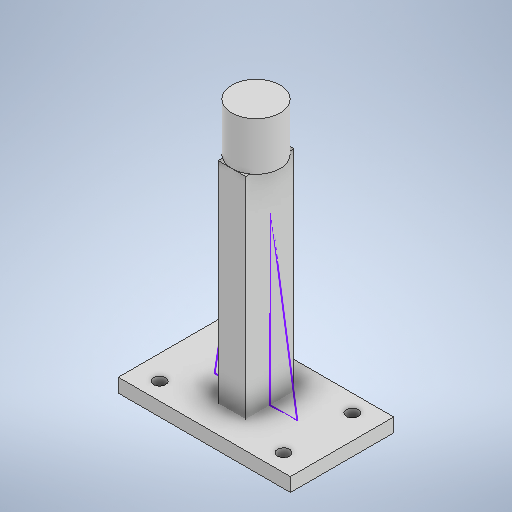
# Autodesk Inventor part: Stuetze_v2
Saved by Autodesk Inventor 2025 (Build 290162000, 162)
## iProperties
Created: 2026-06-23
Part Number: Stuetze_v2
Material: Generisch
Document SubType Name: Modeling
Designer: GemmiDad-GBSE
Density: 1 g/cm^3
Appearance: Vorgabe
Author: GemmiDad-GBSE
Autodesk Inventor part; units mm, degrees
ref_plane "YZ Plane" through (0, 0, 0) normal (1, 0, 0) x (0, 1, 0)
ref_plane "XZ Plane" through (0, 0, 0) normal (0, 1, 0) x (-1, 0, 0)
sketch "Skizze1" plane through (0, 0, 0) normal (0, 0, 1) x (1, 0, 0)
  line L0 (-25, -15) -> (25, -15)
  line L1 (25, -15) -> (25, 15)
  line L2 (25, 15) -> (-25, 15)
  line L3 (-25, 15) -> (-25, -15)
  constraints: 8 end point, 2 parallel, 1 horizontal, 1 perpendicular
extrude "Extrusion1" add sketch "Skizze1" along normal blind 4
sketch "Skizze2" plane through (0, 0, 0) normal (0, 0, 1) x (1, 0, 0)
  line L0 (-4, -7) -> (4, -7)
  line L1 (4, -7) -> (4, 7)
  line L2 (4, 7) -> (-4, 7)
  line L3 (-4, 7) -> (-4, -7)
  constraints: 8 end point, 2 parallel, 1 horizontal, 1 perpendicular
extrude "Extrusion2" add sketch "Skizze2" along normal blind 65 separate body
ref_plane "Arbeitsebene1" through (0, 0, 65) normal (0, 0, 1) x (1, 0, 0)
sketch "Skizze3" plane through (0, 0, 65) normal (0, 0, 1) x (1, 0, 0)
  circle A0 centre (0, 0) radius 7
  constraints: 1 centre point
extrude "Extrusion3" add sketch "Skizze3" along normal blind 14 separate body
sketch "Skizze4" plane through (0, 0, 0) normal (0, 1, 0) x (-1, 0, 0)
  line L0 (4, 4) -> (12, 4)
  line L1 (12, 4) -> (4, 55)
  line L2 (4, 55) -> (4, 4)
  constraints: 6 end point
sketch "Skizze5" plane through (0, 0, 0) normal (0, 1, 0) x (-1, 0, 0)
  line L0 (-4, 4) -> (-12, 4)
  line L1 (-12, 4) -> (-4, 55)
  line L2 (-4, 55) -> (-4, 4)
  constraints: 6 end point
sketch "Skizze6" plane through (0, 0, 0) normal (1, 0, 0) x (0, 1, 0)
  circle A0 centre (0, 72) radius 4.25
  constraints: 1 centre point
extrude "Extrusion4" cut sketch "Skizze6" along normal mid plane 51 bodies 1
sketch "Skizze7" plane through (0, 0, 0) normal (0, 0, 1) x (1, 0, 0)
  circle A0 centre (-18, -10) radius 1.75
  circle A1 centre (-18, 10) radius 1.75
  circle A2 centre (18, -10) radius 1.75
  circle A3 centre (18, 10) radius 1.75
  constraints: 4 centre point
extrude "Extrusion5" cut sketch "Skizze7" along normal blind 5 bodies 1
